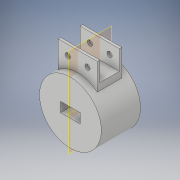
# Autodesk Inventor part: MountV05
Saved by Autodesk Inventor 2019.1 (Build 231200000, 200)
## iProperties
Created: 2018-11-03
Part Number: MountV05
Material: Generic
Document SubType Name: Modeling
Designer: steele
Density: 1 g/cm^3
Appearance: Default
Author: steele
Autodesk Inventor part; units mm, degrees
ref_plane "XZ Plane" through (0, 0, 0) normal (0, 1, 0) x (-1, 0, 0)
ref_plane "XY Plane" through (0, 0, 0) normal (0, 0, 1) x (1, 0, 0)
sketch "Sketch1" plane through (0, 0, 0) normal (0, 0, 1) x (1, 0, 0)
  circle A0 centre (0, 0) radius 40
  dimension "d0" = 80
  constraints: 1 centre point, 1 coincident
  measures "d0" diameter of A0
extrude "Extrusion1" add sketch "Sketch1" along normal blind 50.8
sketch "Sketch2" plane through (0, 0, 0) normal (0, 0, -1) x (-1, 0, 0)
  circle A0 centre (0, 0) radius 31
  circle A1 centre (0, 0) radius 24
  dimension "d3" = 62
  dimension "d4" = 48
  constraints: 2 centre point, 2 coincident
  measures "d3" diameter of A0
  measures "d4" diameter of A1
extrude "Extrusion2" cut sketch "Sketch2" against normal blind 2
sketch "Sketch3" plane through (0, 0, 0) normal (0, 0, -1) x (-1, 0, 0)
  circle A0 centre (0, 0) radius 3.175
  dimension "d25" = 6.35
  constraints: 1 centre point, 1 coincident
  measures "d25" diameter of A0
extrude "Extrusion3" cut sketch "Sketch3" against normal through all
sketch "Sketch4" plane through (0, 0, 50.8) normal (0, 0, 1) x (1, 0, 0)
  line L0 (-12.7, -6.35) -> (12.7, -6.35)
  line L1 (12.7, -6.35) -> (12.7, 6.35)
  line L2 (12.7, 6.35) -> (-12.7, 6.35)
  line L3 (-12.7, 6.35) -> (-12.7, -6.35)
  line L4 (-12.7, -6.35) -> (12.7, 6.35) construction
  line L5 (12.7, -6.35) -> (-12.7, 6.35) construction
  point P0 (0, 0)
  dimension "d28" = 25.4
  dimension "d29" = 12.7
  constraints: 12 end point, 2 midpoint, 2 parallel, 1 horizontal, 1 perpendicular
  measures "d28" distance of L1.end L2.end
  measures "d29" distance of L2.end L0.start
extrude "Extrusion4" cut sketch "Sketch4" against normal through all
sketch "Sketch6" plane through (0, 0, 0) normal (1, 0, 0) x (0, 1, 0)
  line L0 (40, 0) -> (40, 50.8) construction
  line L1 (40, 25.4) -> (-40, 25.4) construction
  line L2 (-40, 0) -> (-40, 50.8) construction
  line L3 (40, 9.525) -> (65.4, 9.525)
  line L4 (65.4, 9.525) -> (65.4, 25.4)
  line L5 (40, 25.4) -> (27.3, 25.4)
  line L6 (27.3, 9.525) -> (40, 9.525)
  line L7 (27.3, 25.4) -> (27.3, 9.525)
  line L8 (40, 41.275) -> (65.4, 41.275)
  line L9 (65.4, 41.275) -> (65.4, 25.4)
  line L10 (27.3, 41.275) -> (40, 41.275)
  line L11 (27.3, 25.4) -> (27.3, 41.275)
  point P0 (0, 0)
  dimension "d34" = 25.4
  dimension "d35" = 12.7
  dimension "d36" = 15.875
  constraints: 20 end point, 3 symmetric about line, 2 midpoint, 2 parallel, 2 point on line, 1 horizontal, 1 perpendicular, 1 vertical
  measures "d34" distance between parallel lines of L4 L0
  measures "d35" distance from line of L7 L1.start
  measures "d36" distance from line of L1.start L3
extrude "Extrusion5" add sketch "Sketch6" along normal mid plane 50.8
sketch "Sketch8" plane through (-25.4, 65.4, 41.275) normal (0, 1, 0) x (1, 0, 0)
  line L0 (0, 31.75) -> (50.8, 31.75) projected
  line L1 (0, 3.175) -> (50.8, 3.175)
  line L2 (50.8, 3.175) -> (50.8, 28.575)
  line L3 (50.8, 28.575) -> (0, 28.575)
  line L4 (0, 28.575) -> (0, 3.175)
  line L5 (0, 3.175) -> (50.8, 28.575) construction
  line L6 (50.8, 3.175) -> (0, 28.575) construction
  point P0 (25.4, 41.275)
  point P1 (25.4, 15.875)
  dimension "d43" = 15.875
  dimension "d44" = 25.4
  constraints: 12 end point, 2 midpoint, 2 parallel, 1 horizontal, 1 perpendicular
  measures "d43" distance from line of point (25.4, 15.875) L0
  measures "d44" distance of L2.end L1.end
extrude "Extrusion7" cut sketch "Sketch8" against normal blind 25.4
sketch "Sketch9" plane through (0, 0, 41.275) normal (0, 0, 1) x (1, 0, 0)
  line L0 (-25.4, 65.4) -> (25.4, 65.4) projected
  line L1 (0, 86.48) -> (0, -61.08) projected
  point P0 (0, 0)
  point P1 (-12.7, 52.7)
  point P2 (12.7, 52.7)
  dimension "d47" = 12.7
  dimension "d48" = 12.7
  dimension "d49" = 12.7
  dimension "d50" = 12.7
  measures "d47" distance from line of point (-12.7, 52.7) L0
  measures "d48" distance from line of point (12.7, 52.7) L0
  measures "d49" distance from line of point (-12.7, 52.7) L1
  measures "d50" distance from line of point (12.7, 52.7) L1
hole "Hole1" at (-12.7, 52.7, 41.275) at (12.7, 52.7, 41.275) direction (0, 0, -1) diameter 6.7564 end through all clearance for "Hex Machine Screw" size "1/4" standard "Ansi Unified Screw Threads"
equation "\"d0\" = mountOuterDiameter"
equation "\"d3\" = ringOuterDiam + ringDiamGap"
equation "\"d4\" = ringInnerDiam - ringDiamGap"
equation "\"ringOuterDiam\" = 60"
equation "\"ringInnerDiam\" = 50"
equation "\"ringThickness\" = 1.5"
equation "\"ringDiamGap\" = 2"
equation "\"mountOuterDiameter\" = 80"
body "Solid1"
